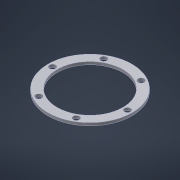
# Autodesk Inventor part: P022-Joint_carter_bouchon_vilbrequin
Saved by Autodesk Inventor 2021.3 (Build 253353000, 353)
## iProperties
Created: 2022-06-06
Part Number: P022-Joint_carter_bouchon_vilbrequin
Material: Polytetrafluoroethylene
Document SubType Name: Modeling
Designer: Rémi Heredero
Density: 2.02 g/cm^3
Appearance: PTFE
Author: Rémi Heredero
Autodesk Inventor part; units mm, degrees
ref_plane "YZ Plane" through (0, 0, 0) normal (1, 0, 0) x (0, 1, 0)
ref_plane "XZ Plane" through (0, 0, 0) normal (0, 1, 0) x (-1, 0, 0)
ref_plane "XY Plane" through (0, 0, 0) normal (0, 0, 1) x (1, 0, 0)
sketch "Sketch2" plane through (0, 0, 0) normal (0, 0, 1) x (1, 0, 0)
  circle A0 centre (0, 0) radius 30
  circle A1 centre (0, 0) radius 23.5
  dimension "d0" = 60
  dimension "d1" = 47
  constraints: 2 centre point, 2 coincident
  measures "d0" diameter of A0
  measures "d1" diameter of A1
extrude "Extrusion1" add sketch "Sketch2" along normal blind 2
sketch "Sketch3" plane through (0, 0, 0) normal (0, 0, -1) x (-1, 0, 0)
  circle A0 centre (-13.375, 23.1662) radius 2.25 projected
  circle A1 centre (-13.375, -23.1662) radius 2.25 projected
  circle A2 centre (26.75, 0) radius 2.25 projected
  circle A3 centre (13.375, -23.1662) radius 2.25 projected
  circle A4 centre (-26.75, 0) radius 2.25 projected
  circle A5 centre (13.375, 23.1662) radius 2.25 projected
  circle A6 centre (0, 0) radius 30 construction
  point P0 (0, 0)
hole "Hole1" at (-13.375, 23.1662, 0) at (-26.75, 0, 0) at (-13.375, -23.1662, 0) at (13.375, -23.1662, 0) at (26.75, 0, 0) at (13.375, 23.1662, 0) direction (0, 0, 1) diameter 4.5 end through all start extended yes clearance for "Countersunk Flat Head Screw ISO 2009/7046" size "M4" standard "ISO"
body "Solid1"
